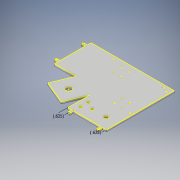
# Autodesk Inventor part: Cut1
Saved by Autodesk Inventor 2018 (Build 220112000, 112)
## iProperties
Created: 2018-10-20
Part Number: Cut1
Material: Generic
Document SubType Name: Modeling
Designer: jpark
Density: 1 g/cm^3
Appearance: Default
Author: jpark
Autodesk Inventor part; units mm, degrees
ref_plane "YZ Plane" through (0, 0, 0) normal (1, 0, 0) x (0, 1, 0)
ref_plane "XZ Plane" through (0, 0, 0) normal (0, 1, 0) x (-1, 0, 0)
ref_plane "XY Plane" through (0, 0, 0) normal (0, 0, 1) x (1, 0, 0)
sketch "Sketch1" plane through (0, 0, 0) normal (0, 1, 0) x (-1, 0, 0)
  line L0 (0, 0) -> (0, -152.4)
  line L1 (0, -152.4) -> (203.2, -152.4)
  line L2 (203.2, -152.4) -> (203.2, -31.75)
  line L3 (203.2, -31.75) -> (127, 0)
  line L4 (127, 0) -> (0, 0)
  dimension "d0" = 203.2
  dimension "d1" = 120.65
  dimension "d2" = 127
  dimension "d3" = 152.4
  constraints: 10 end point, 2 perpendicular, 1 parallel, 1 vertical
  measures "d0" distance of L0.end L1.end
  measures "d1" distance of L1.end L2.end
  measures "d2" distance of L3.end L0.start
  measures "d3" distance of L0.start L0.end
extrude "Extrusion1" add sketch "Sketch1" along normal blind 6.35
sketch "Sketch3" plane through (-127, 0, 0) normal (0, 0, 1) x (1, 0, 0)
  line L0 (0, 0) -> (127, 0) projected
  line L1 (127, 0) -> (127, 6.35) projected
  line L2 (0, 6.35) -> (127, 6.35) projected
  line L3 (0, 0) -> (0, 6.35) projected
extrude "Extrusion2" add sketch "Sketch3" along normal blind 71.12
sketch "Sketch4" plane through (-203.2, 0, -31.75) normal (-0.3846, 0, 0.9231) x (0.9231, 0, 0.3846)
  line L0 (0, 0) -> (82.55, 0) projected
  line L1 (82.55, 0) -> (82.55, 6.35) projected
  line L2 (0, 6.35) -> (82.55, 6.35) projected
  line L3 (0, 0) -> (0, 6.35) projected
  point P0 (199.7808, 0)
extrude "Extrusion3" add sketch "Sketch4" along normal blind 71.12
sketch "Sketch5" plane through (-203.2, 0, -152.4) normal (-1, 0, 0) x (0, 0, 1)
  line L0 (0, 0) -> (120.65, 0) projected
  line L1 (120.65, 0) -> (120.65, 6.35) projected
  line L2 (0, 6.35) -> (120.65, 6.35) projected
  line L3 (0, 0) -> (0, 6.35) projected
  point P0 (152.4, 0)
extrude "Extrusion4" add sketch "Sketch5" along normal blind 71.12
sketch "Sketch7" plane through (0, 6.35, 0) normal (0, 1, 0) x (1, 0, 0)
  line L0 (0, -71.12) -> (-127, -71.12) projected
  line L1 (-12.7, -71.12) -> (-19.05, -71.12)
  line L2 (-19.05, -71.12) -> (-19.05, -83.82)
  line L3 (-19.05, -83.82) -> (-12.7, -83.82)
  line L4 (-12.7, -83.82) -> (-12.7, -71.12)
  circle A0 centre (-15.875, -80.645) radius 1.397
  line L5 (0, 152.4) -> (0, -71.12) projected
  line L6 (-107.95, -71.12) -> (-114.3, -71.12)
  line L7 (-114.3, -71.12) -> (-114.3, -83.82)
  line L8 (-114.3, -83.82) -> (-107.95, -83.82)
  line L9 (-107.95, -83.82) -> (-107.95, -71.12)
  circle A1 centre (-111.125, -80.645) radius 1.397
  line L10 (-127, 0) -> (-127, -71.12) projected
  point P0 (0, 0)
  dimension "d13" = 12.7
  dimension "d14" = 6.35
  dimension "d15" = 2.794
  dimension "d16" = 3.175
  dimension "d17" = 12.7
  dimension "d18" = 3.175
  dimension "d19" = 12.7
  dimension "d20" = 6.35
  dimension "d21" = 2.794
  dimension "d22" = 3.175
  dimension "d23" = 3.175
  dimension "d24" = 0
  dimension "d25" = 12.7
  constraints: 16 end point, 4 parallel, 2 centre point, 2 horizontal, 2 perpendicular, 1 point on line
  measures "d13" distance of L1.end L2.end
  measures "d14" distance of L2.end L3.end
  measures "d15" diameter of A0
  measures "d16" distance from line of L3 A0.centre
  measures "d17" distance between parallel lines of L5 L4
  measures "d18" distance from line of L4 A0.centre
  measures "d19" distance of L6.end L7.end
  measures "d20" distance of L7.end L8.end
  measures "d21" diameter of A1
  measures "d22" distance from line of L8 A1.centre
  measures "d23" distance from line of L9 A1.centre
  measures "d24" distance between parallel lines of L6 L0
  measures "d25" distance between parallel lines of L10 L7
extrude "Extrusion5" add sketch "Sketch7" against normal blind 6.35
sketch "Sketch8" plane through (0, 6.35, 0) normal (0, 1, 0) x (1, 0, 0)
  line L0 (-274.32, 152.4) -> (-274.32, 31.75) projected
  line L1 (-274.32, 44.45) -> (-287.02, 44.45)
  line L2 (-287.02, 44.45) -> (-287.02, 50.8)
  line L3 (-287.02, 50.8) -> (-274.32, 50.8)
  line L4 (-274.32, 50.8) -> (-274.32, 44.45)
  line L5 (-203.2, 31.75) -> (-274.32, 31.75) projected
  circle A0 centre (-283.845, 47.625) radius 1.397
  line L6 (-274.32, 133.35) -> (-287.02, 133.35)
  line L7 (-287.02, 133.35) -> (-287.02, 139.7)
  line L8 (-287.02, 139.7) -> (-274.32, 139.7)
  line L9 (-274.32, 139.7) -> (-274.32, 133.35)
  circle A1 centre (-283.845, 136.525) radius 1.397
  line L10 (0, 152.4) -> (-274.32, 152.4) projected
  point P0 (0, 0)
  point P1 (-272.7325, 33.3375)
  dimension "d33" = 6.35
  dimension "d34" = 12.7
  dimension "d35" = 12.7
  dimension "d36" = 2.794
  dimension "d37" = 3.175
  dimension "d38" = 3.175
  dimension "d39" = 6.35
  dimension "d40" = 12.7
  dimension "d41" = 2.794
  dimension "d42" = 3.175
  dimension "d43" = 3.175
  dimension "d44" = 0
  dimension "d45" = 12.7
  constraints: 16 end point, 4 parallel, 2 centre point, 2 horizontal, 2 perpendicular, 1 point on line
  measures "d33" distance of L1.end L2.end
  measures "d34" distance of L2.end L3.end
  measures "d35" distance between parallel lines of L1 L5
  measures "d36" diameter of A0
  measures "d37" distance from line of L1 A0.centre
  measures "d38" distance from line of L2 A0.centre
  measures "d39" distance of L6.end L7.end
  measures "d40" distance of L7.end L8.end
  measures "d41" diameter of A1
  measures "d42" distance from line of L6 A1.centre
  measures "d43" distance from line of L7 A1.centre
  measures "d44" distance between parallel lines of L0 L9
  measures "d45" distance between parallel lines of L10 L8
extrude "Extrusion6" add sketch "Sketch8" against normal blind 6.35
sketch "Sketch9" plane through (0, 6.35, 0) normal (0, 1, 0) x (1, 0, 0)
  circle A0 centre (-38.1, 19.05) radius 1.397
  circle A1 centre (-63.5, 19.05) radius 1.397
  circle A2 centre (-38.1, 44.45) radius 1.397
  circle A3 centre (-63.5, 44.45) radius 1.397
  circle A4 centre (-127.2575, 106.1211) radius 1.397
  circle A5 centre (-152.6575, 106.1211) radius 1.397
  circle A6 centre (-127.2575, 131.5211) radius 1.397
  circle A7 centre (-152.6575, 131.5211) radius 1.397
  point P0 (0, 0)
  point P1 (-127, 0)
  dimension "d48" = 2.794
  dimension "d49" = 2.794
  dimension "d50" = 2.794
  dimension "d51" = 2.794
  dimension "d52" = 25.4
  dimension "d53" = 25.4
  dimension "d54" = 25.4
  dimension "d55" = 25.4
  dimension "d56" = 25.4
  dimension "d57" = 25.4
  dimension "d58" = 19.05
  dimension "d59" = 38.1
  dimension "d60" = 2.794
  dimension "d61" = 2.794
  dimension "d62" = 2.794
  dimension "d63" = 2.794
  dimension "d64" = 25.4
  dimension "d65" = 25.4
  dimension "d66" = 25.4
  dimension "d67" = 25.4
  dimension "d68" = 25.4
  dimension "d69" = 25.4
  constraints: 8 centre point
  measures "d48" diameter of A0
  measures "d49" diameter of A1
  measures "d50" diameter of A2
  measures "d51" diameter of A3
  measures "d52" distance of A3.centre A1.centre
  measures "d53" distance of A3.centre A2.centre
  measures "d54" horizontal distance of A1.centre A2.centre
  measures "d55" distance of A1.centre A0.centre
  measures "d56" horizontal distance of A3.centre A0.centre
  measures "d57" horizontal distance of A1.centre A2.centre
  measures "d58" vertical distance of A1.centre point (-127, 0)
  measures "d59" horizontal distance of point (0, 0) A0.centre
  measures "d60" diameter of A4
  measures "d61" diameter of A5
  measures "d62" diameter of A6
  measures "d63" diameter of A7
  measures "d64" distance of A7.centre A5.centre
  measures "d65" distance of A7.centre A6.centre
  measures "d66" horizontal distance of A5.centre A6.centre
  measures "d67" distance of A5.centre A4.centre
  measures "d68" horizontal distance of A7.centre A4.centre
  measures "d69" horizontal distance of A5.centre A6.centre
extrude "Extrusion7" cut sketch "Sketch9" against normal blind 6.35
sketch "Sketch10" plane through (0, 6.35, 0) normal (0, 1, 0) x (1, 0, 0)
  circle A0 centre (-9.271, 15.875) radius 1.524
  circle A1 centre (-9.271, 136.525) radius 1.524
  line L0 (0, 152.4) -> (-274.32, 152.4) projected
  circle A2 centre (-283.845, 47.625) radius 1.397 projected
  circle A3 centre (-283.845, 136.525) radius 1.397 projected
  line L1 (0, 152.4) -> (0, -71.12) projected
  circle A4 centre (-25.4, 143.129) radius 1.524
  circle A5 centre (-190.5, 143.129) radius 1.524
  point P0 (0, 0)
  point P1 (-203.2, 31.75)
  dimension "d72" = 3.048
  dimension "d73" = 3.048
  dimension "d74" = 15.875
  dimension "d75" = 120.65
  dimension "d76" = 9.271
  dimension "d77" = 9.271
  dimension "d78" = 3.048
  dimension "d79" = 3.048
  dimension "d80" = 9.271
  dimension "d81" = 25.4
  dimension "d82" = 12.7
  dimension "d83" = 9.271
  dimension "d101" = 88.9
  constraints: 4 centre point
  measures "d72" diameter of A0
  measures "d73" diameter of A1
  measures "d74" distance from line of L0 A1.centre
  measures "d75" distance of A1.centre A0.centre
  measures "d76" distance from line of L1 A1.centre
  measures "d77" horizontal distance of L0.start A0.centre
  measures "d78" diameter of A4
  measures "d79" diameter of A5
  measures "d80" distance from line of L0 A4.centre
  measures "d81" distance from line of L1 A4.centre
  measures "d82" horizontal distance of point (-203.2, 31.75) A5.centre
  measures "d83" distance from line of L0 A5.centre
  measures "d101" distance of A2.centre A3.centre
extrude "Extrusion8" cut sketch "Sketch10" against normal blind 6.35 contours A0 | A1 | A4 | A5
sketch "Sketch11" plane through (0, 6.35, 0) normal (0, 1, 0) x (1, 0, 0)
  circle A0 centre (-178.7769, -16.9496) radius 8.763
  circle A1 centre (-107.95, -48.26) radius 4.2545
  circle A2 centre (-82.55, -35.56) radius 4.2545
  circle A3 centre (-107.95, -22.86) radius 4.2545
  line L0 (-19.05, -71.12) -> (-107.95, -71.12) projected
  line L1 (-127, 0) -> (-154.3538, -65.6492) projected
  line L2 (-127, 0) -> (-127, -71.12) projected
  line L3 (-154.3538, -65.6492) -> (-230.5538, -33.8992) projected
  point P0 (0, 0)
  dimension "d86" = 8.509
  dimension "d87" = 8.509
  dimension "d88" = 8.509
  dimension "d89" = 17.526
  dimension "d90" = 22.86
  dimension "d91" = 22.86
  dimension "d92" = 35.56
  dimension "d93" = 44.45
  dimension "d94" = 19.05
  dimension "d95" = 19.05
  constraints: 4 centre point, 1 other
  measures "d86" diameter of A1
  measures "d87" diameter of A2
  measures "d88" diameter of A3
  measures "d89" diameter of A0
  measures "d90" distance from line of L0 A1.centre
  measures "d91" vertical distance of L1.start A3.centre
  measures "d92" distance from line of A2.centre L0
  measures "d93" distance from line of L2 A2.centre
  measures "d94" distance from line of L2 A1.centre
  measures "d95" distance from line of A3.centre L2
extrude "Extrusion9" cut sketch "Sketch11" against normal blind 6.35
sketch "Sketch12" plane through (0, 6.35, 0) normal (0, 1, 0) x (1, 0, 0)
  circle A0 centre (-36.1734, -35.56) radius 6.35
  line L0 (0, 152.4) -> (0, -71.12) projected
  line L1 (-127, 0) -> (-127, -71.12) projected
  point P0 (0, 0)
  dimension "d98" = 12.7
  constraints: 1 centre point, 1 other
  measures "d98" diameter of A0
extrude "Extrusion10" cut sketch "Sketch12" against normal blind 6.35
sketch "Sketch13" plane through (0, 6.35, 0) normal (0, 1, 0) x (1, 0, 0)
  line L0 (0, 152.4) -> (-274.32, 152.4) projected
  line L1 (0, 152.4) -> (0, -71.12) projected
  circle A0 centre (-36.1734, -35.56) radius 6.35 projected
  circle A1 centre (-107.95, -22.86) radius 4.2545 projected
  circle A2 centre (-107.95, -48.26) radius 4.2545 projected
  circle A3 centre (-82.55, -35.56) radius 4.2545 projected
  circle A4 centre (-178.7769, -16.9496) radius 8.763 projected
  circle A5 centre (-25.4, 143.129) radius 1.524 projected
  circle A6 centre (-9.271, 15.875) radius 1.524 projected
  circle A7 centre (-9.271, 136.525) radius 1.524 projected
  circle A8 centre (-190.5, 143.129) radius 1.524 projected
  circle A9 centre (-127.2575, 131.5211) radius 1.397 projected
  circle A10 centre (-127.2575, 106.1211) radius 1.397 projected
  circle A11 centre (-38.1, 44.45) radius 1.397 projected
  circle A12 centre (-38.1, 19.05) radius 1.397 projected
  circle A13 centre (-63.5, 19.05) radius 1.397 projected
  circle A14 centre (-63.5, 44.45) radius 1.397 projected
  circle A15 centre (-152.6575, 106.1211) radius 1.397 projected
  circle A16 centre (-152.6575, 131.5211) radius 1.397 projected
  circle A17 centre (-283.845, 47.625) radius 1.397 projected
  circle A18 centre (-283.845, 136.525) radius 1.397 projected
  circle A19 centre (-15.875, -80.645) radius 1.397 projected
  circle A20 centre (-111.125, -80.645) radius 1.397 projected
  line L2 (0, 152.4) -> (0, -71.12) projected
  line L3 (0, 152.4) -> (-274.32, 152.4) projected
  line L4 (-274.32, 139.7) -> (-274.32, 152.4) projected
  line L5 (-287.02, 139.7) -> (-274.32, 139.7) projected
  line L6 (-287.02, 133.35) -> (-287.02, 139.7) projected
  line L7 (-274.32, 133.35) -> (-287.02, 133.35) projected
  line L8 (-274.32, 50.8) -> (-274.32, 133.35) projected
  line L9 (-287.02, 50.8) -> (-274.32, 50.8) projected
  line L10 (-287.02, 44.45) -> (-287.02, 50.8) projected
  line L11 (-274.32, 44.45) -> (-287.02, 44.45) projected
  line L12 (-274.32, 31.75) -> (-274.32, 44.45) projected
  line L13 (-203.2, 31.75) -> (-274.32, 31.75) projected
  line L14 (-203.2, 31.75) -> (-230.5538, -33.8992) projected
  line L15 (-154.3538, -65.6492) -> (-230.5538, -33.8992) projected
  line L16 (-127, 0) -> (-154.3538, -65.6492) projected
  line L17 (-127, 0) -> (-127, -71.12) projected
  line L18 (-114.3, -71.12) -> (-127, -71.12) projected
  line L19 (-114.3, -71.12) -> (-114.3, -83.82) projected
  line L20 (-114.3, -83.82) -> (-107.95, -83.82) projected
  line L21 (-107.95, -83.82) -> (-107.95, -71.12) projected
  line L22 (-19.05, -71.12) -> (-107.95, -71.12) projected
  line L23 (-19.05, -71.12) -> (-19.05, -83.82) projected
  line L24 (-19.05, -83.82) -> (-12.7, -83.82) projected
  line L25 (-12.7, -83.82) -> (-12.7, -71.12) projected
  line L26 (0, -71.12) -> (-12.7, -71.12) projected
  point P0 (0, 0)
  dimension "d102" = 15.875
  dimension "d103" = 15.875
  measures "d102" horizontal distance of L17.end A20.centre
  measures "d103" horizontal distance of L1.end A19.centre
body "Solid1"
